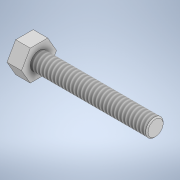
# Autodesk Inventor part: Screw
Saved by Autodesk Inventor 2022 (Build 260153000, 153)
## iProperties
Created: 2022-08-20
Part Number: Screw
Material: Generic
Document SubType Name: Modeling
Designer: yashm
Density: 1 g/cm^3
Appearance: Default
Author: yashm
Autodesk Inventor part; units mm, degrees
ref_plane "YZ Plane" through (0, 0, 0) normal (1, 0, 0) x (0, 1, 0)
ref_plane "XZ Plane" through (0, 0, 0) normal (0, 1, 0) x (-1, 0, 0)
ref_plane "XY Plane" through (0, 0, 0) normal (0, 0, 1) x (1, 0, 0)
sketch "Sketch1" plane through (0, 0, 0) normal (1, 0, 0) x (0, 1, 0)
  line L0 (11.1677, 16.6703) -> (5.9715, 19.6703)
  line L1 (5.9715, 19.6703) -> (0.7754, 16.6703)
  line L2 (0.7754, 16.6703) -> (0.7754, 10.6703)
  line L3 (0.7754, 10.6703) -> (5.9715, 7.6703)
  line L4 (5.9715, 7.6703) -> (11.1677, 10.6703)
  line L5 (11.1677, 10.6703) -> (11.1677, 16.6703)
  point P0 (0, 0)
  dimension "d0" = 120
  dimension "d1" = 120
  dimension "d2" = 6
  constraints: 12 end point, 4 equal length, 2 parallel, 1 vertical
  measures "d0" angle of L4 L5
  measures "d1" angle of L5 L0
  measures "d2" distance of L4.end L0.start
extrude "Extrusion1" add sketch "Sketch1" along normal blind 5
sketch "Sketch2" plane through (5, 0, 0) normal (1, 0, 0) x (0, 0, -1)
  circle A0 centre (-13.6703, 5.9715) radius 3
  point P0 (0, 0)
  point P1 (-16.6703, 11.1677)
  point P2 (-10.6703, 0.7754)
  point P3 (-16.6703, 0.7754)
  dimension "d5" = 6
  dimension "d6" = 6
  dimension "d7" = 6
  constraints: 1 centre point
  measures "d5" diameter of A0
  measures "d6" distance of A0.centre point (-16.67, 11.168)
  measures "d7" distance of point (-16.67, 0.775) A0.centre
extrude "Extrusion2" add sketch "Sketch2" along normal blind 40
thread "Thread1" size "1/4-20 UNC" class "2A" standard "ANSI Unified Screw Threads" full length
chamfer "Chamfer1" distance 0.4 angle 45 1 edges at (45, 5.9715, 16.6703)
body "Solid1"
